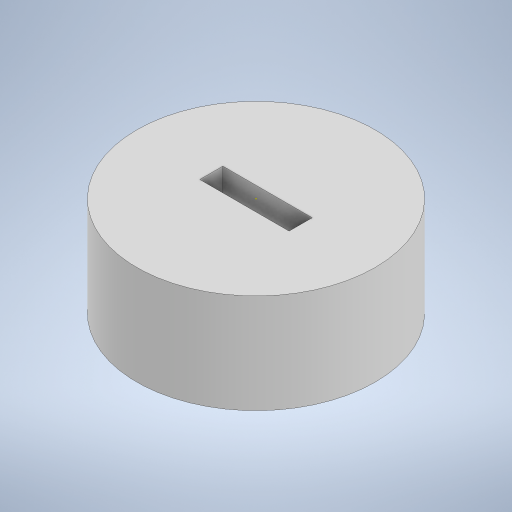
# Autodesk Inventor part: Sendok 1
Saved by Autodesk Inventor 2024 (Build 280153000, 153)
## iProperties
Created: 2023-10-30
Part Number: Sendok 1
Material: Generic
Document SubType Name: Modeling
Designer: lazy1
Density: 1 g/cm^3
Appearance: Default
Author: lazy1
Autodesk Inventor part; units mm, degrees
ref_plane "YZ Plane" through (0, 0, 0) normal (1, 0, 0) x (0, 1, 0)
ref_plane "XZ Plane" through (0, 0, 0) normal (0, 1, 0) x (-1, 0, 0)
ref_plane "XY Plane" through (0, 0, 0) normal (0, 0, 1) x (1, 0, 0)
sketch "Sketch1" plane through (0, 0, 0) normal (0, 1, 0) x (-1, 0, 0)
  circle A0 centre (0, 0) radius 15
  circle A1 centre (0, 0) radius 2.45
  line L0 (0, 0) -> (8, 0)
  circle A2 centre (8, 0) radius 2.45
  line L1 (8, 0) -> (8, -8)
  line L2 (8, 0) -> (8, 8)
  circle A3 centre (8, 8) radius 2.45
  circle A4 centre (8, -8) radius 2.45
  circle A5 centre (0, 8) radius 2.45
  circle A6 centre (0, -8) radius 2.45
  line L3 (0, 0) -> (-8, 0)
  line L4 (0, 0) -> (8, 0) construction
  circle A7 centre (-8, 0) radius 2.45
  circle A8 centre (-8, -8) radius 2.45
  circle A9 centre (-8, 8) radius 2.45
  circle A10 centre (0, -15) radius 1.25
  circle A11 centre (-15, 0) radius 1.25
  circle A12 centre (0, 15) radius 1.25
  circle A13 centre (15, 0) radius 1.25
  circle A14 centre (0, 0) radius 18
  dimension "d0" = 30
  dimension "d1" = 4.9
  dimension "d2" = 8
  dimension "d3" = 4.9
  dimension "d4" = 8
  dimension "d5" = 8
  dimension "d6" = 4.9
  dimension "d7" = 4.9
  dimension "d8" = 4.9
  dimension "d9" = 4.9
  dimension "d10" = 8
  dimension "d11" = 180
  dimension "d12" = 4.9
  dimension "d13" = 4.9
  dimension "d14" = 4.9
  dimension "d15" = 2.5
  dimension "d16" = 2.5
  dimension "d17" = 2.5
  dimension "d18" = 2.5
  dimension "d19" = 36
  constraints: 15 centre point, 10 end point, 7 coincident, 4 point on circle, 3 horizontal, 2 vertical, 1 collinear
  measures "d0" diameter of A0
  measures "d1" diameter of A1
  measures "d2" distance of L0.start L0.end
  measures "d3" diameter of A2
  measures "d4" distance of L1.start L1.end
  measures "d5" distance of L1.start L2.end
  measures "d6" diameter of A3
  measures "d7" diameter of A4
  measures "d8" diameter of A5
  measures "d9" diameter of A6
  measures "d10" distance of L0.start L3.end
  measures "d11" angle of L3 L4
  measures "d12" diameter of A7
  measures "d13" diameter of A8
  measures "d14" diameter of A9
  measures "d15" diameter of A10
  measures "d16" diameter of A11
  measures "d17" diameter of A12
  measures "d18" diameter of A13
  measures "d19" diameter of A14
extrude "Extrusion1" add sketch "Sketch1" along normal blind 10 contours A13 A0 A10 A11 A12 | A14
sketch "Sketch2" plane through (0, 10, 0) normal (0, 1, 0) x (1, 0, 0)
  circle A0 centre (0, 0) radius 18
  dimension "d24" = 36
  constraints: 1 centre point, 1 coincident
  measures "d24" diameter of A0
extrude "Extrusion2" add sketch "Sketch2" along normal blind 5
sketch "Sketch3" plane through (0, 15, 0) normal (0, 1, 0) x (1, 0, 0)
  point P0 (0, 0)
sketch "Sketch4" plane through (0, 15, 0) normal (0, 1, 0) x (1, 0, 0)
  line L0 (-6.75, 1.75) -> (6.75, 1.75)
  line L1 (6.75, 1.75) -> (6.75, -1.75)
  line L2 (6.75, -1.75) -> (-6.75, -1.75)
  line L3 (-6.75, -1.75) -> (-6.75, 1.75)
  line L4 (-6.75, 1.75) -> (6.75, -1.75) construction
  line L5 (6.75, 1.75) -> (-6.75, -1.75) construction
  point P0 (0, 0)
  dimension "d25" = 13.5
  dimension "d26" = 3.5
  constraints: 12 end point, 2 midpoint, 2 parallel, 1 horizontal, 1 perpendicular
  measures "d25" distance of L1.end L2.end
  measures "d26" distance of L0.end L1.end
extrude "Extrusion3" cut sketch "Sketch4" against normal blind 15
body "Solid1"
